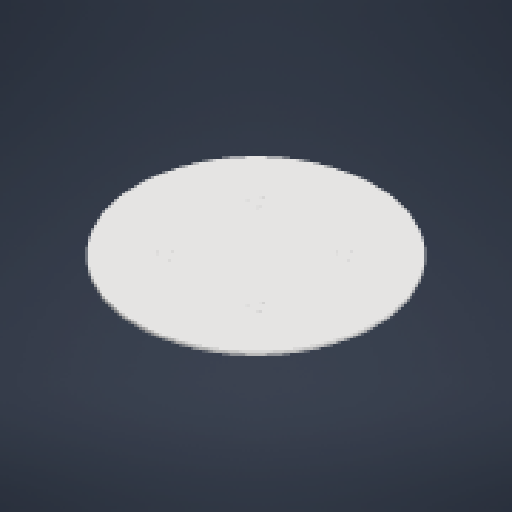
# Autodesk Inventor part: Base
Saved by Autodesk Inventor 2023 (Build 270158000, 158)
## iProperties
Created: 2023-10-25
Part Number: Base
Material: Generic
Document SubType Name: Modeling
Designer: Abhinav
Density: 1 g/cm^3
Appearance: Default
Author: Abhinav
Autodesk Inventor part; units mm, degrees
ref_plane "YZ Plane" through (0, 0, 0) normal (1, 0, 0) x (0, 1, 0)
ref_plane "XZ Plane" through (0, 0, 0) normal (0, 1, 0) x (-1, 0, 0)
ref_plane "XY Plane" through (0, 0, 0) normal (0, 0, 1) x (1, 0, 0)
sketch "Sketch1" plane through (0, 0, 0) normal (0, 1, 0) x (-1, 0, 0)
  circle A0 centre (0, 0) radius 200
  circle A1 centre (-62.1988, 52) radius 1.5
  circle A2 centre (-71.7439, 67.4891) radius 1.5
  circle A3 centre (-62.5, 62.5) radius 13.5 construction
  circle A4 centre (-53.5573, 68.0109) radius 1.5
  circle A5 centre (53.2561, 67.4891) radius 1.5
  circle A6 centre (62.8012, 52) radius 1.5
  circle A7 centre (71.4427, 68.0109) radius 1.5
  circle A8 centre (62.5, 62.5) radius 13.5 construction
  circle A9 centre (53.2561, -57.5109) radius 1.5
  circle A10 centre (62.8012, -73) radius 1.5
  circle A11 centre (71.4427, -56.9891) radius 1.5
  circle A12 centre (62.5, -62.5) radius 13.5 construction
  circle A13 centre (-71.7439, -57.5109) radius 1.5
  circle A14 centre (-62.1988, -73) radius 1.5
  circle A15 centre (-53.5573, -56.9891) radius 1.5
  circle A16 centre (-62.5, -62.5) radius 13.5 construction
  line L0 (-62.5, 62.5) -> (62.5, 62.5)
  line L1 (62.5, 62.5) -> (62.5, -62.5)
  line L2 (62.5, -62.5) -> (-62.5, -62.5)
  line L3 (-62.5, -62.5) -> (-62.5, 62.5)
  line L4 (-62.5, 62.5) -> (62.5, -62.5) construction
  line L5 (62.5, 62.5) -> (-62.5, -62.5) construction
  point P0 (-62.5, 62.5)
  point P1 (-62.5, 62.5)
  point P2 (-62.5, 62.5)
  point P3 (62.5, 62.5)
  point P4 (62.5, 62.5)
  point P5 (62.5, 62.5)
  point P6 (62.5, -62.5)
  point P7 (62.5, -62.5)
  point P8 (62.5, -62.5)
  point P9 (-62.5, -62.5)
  point P10 (-62.5, -62.5)
  point P11 (-62.5, -62.5)
  dimension "d0" = 400
  dimension "d5" = 125
  constraints: 17 centre point, 12 end point, 2 midpoint, 2 parallel, 2 perpendicular, 1 horizontal, 1 other
  measures "d0" diameter of A0
  measures "d5" distance of L0.end L1.end
extrude "Extrusion1" add sketch "Sketch1" along normal blind 5 contours A0 | A1 L3 L0 L1 A6 L2
body "Solid1"
